Autodesk Fusion 360 part; units mm, degrees
(part 2 of 2)
sketch "Sketch2" plane through (0, 0, 0) normal (0, 0, 1) x (1, 0, 0)
  line L0 (-12.5938, 18.225) -> (358.4062, 18.225)
  line L1 (358.4062, 18.225) -> (358.4062, -133.775)
  line L2 (358.4062, -133.775) -> (-12.5938, -133.775)
  line L3 (-12.5938, -133.775) -> (-12.5938, 18.225)
  line L4 (5.4062, -111.775) -> (18.4063, -111.775)
  line L5 (4.9062, -98.275) -> (4.9062, -111.275)
  dimension "d1" = 371
  dimension "d2" = 152
  dimension "d3" = 22
  dimension "d4" = 17.5
  constraint horizontal L0
  constraint vertical L1
  constraint horizontal L2
  constraint vertical L3
  measures "d1" distance of L0.start L0.end
  measures "d2" distance of L0.start L2.end
  measures "d3" distance of L2 L4
  measures "d4" distance of L3 L5
sketch "Sketch3" plane through (0, 0, 0) normal (0, 0, 1) x (1, 0, 0)
  circle A0 centre (353.4062, 13.225) radius 1.7
  line L0 (-12.5938, 18.225) -> (358.4062, 18.225)
  line L1 (358.4062, 18.225) -> (358.4062, -133.775)
  circle A1 centre (-7.5937, 13.225) radius 1.7
  line L2 (-12.5938, -133.775) -> (-12.5938, 18.225)
  circle A2 centre (-7.5938, -128.775) radius 1.7
  line L3 (358.4062, -133.775) -> (-12.5938, -133.775)
  circle A3 centre (353.4062, -128.775) radius 1.7
  circle A4 centre (-7.5938, 13.225) radius 3
  circle A5 centre (353.4062, 13.225) radius 3
  circle A6 centre (353.4062, -128.775) radius 3
  circle A7 centre (-7.5937, -128.775) radius 3
  dimension "d5" = 3.4
  dimension "d6" = 5
  dimension "d7" = 5
  dimension "d8" = 3.4
  dimension "d9" = 5
  dimension "d10" = 5
  dimension "d11" = 3.4
  dimension "d12" = 5
  dimension "d13" = 5
  dimension "d14" = 3.4
  dimension "d15" = 5
  dimension "d16" = 5
  dimension "d17" = 6
  dimension "d18" = 6
  dimension "d19" = 6
  dimension "d20" = 6
  constraint coincident A1.centre A4.centre
  constraint coincident A2.centre A7.centre
  constraint coincident A3.centre A6.centre
  constraint coincident A0.centre A5.centre
  measures "d5" diameter of A0
  measures "d6" distance of A0.centre L0
  measures "d7" distance of A0.centre L1
  measures "d8" diameter of A1
  measures "d9" distance of A1.centre L2
  measures "d10" distance of L0 A1.centre
  measures "d11" diameter of A2
  measures "d12" distance of A2.centre L3
  measures "d13" distance of L2 A2.centre
  measures "d14" diameter of A3
  measures "d15" distance of L3 A3.centre
  measures "d16" distance of L1 A3.centre
  measures "d17" diameter of A4
  measures "d18" diameter of A5
  measures "d19" diameter of A6
  measures "d20" diameter of A7
extrude "Extrude1" add sketch "Sketch3" along normal blind 1.5 contours L0 L1 L2 L3
extrude "Extrude2" cut sketch "plate-2026-01-22T00_34_46.063Z" along normal blind 1.5
